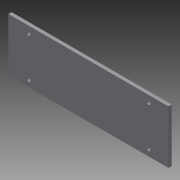
# Autodesk Inventor part: Pneumatic Piston Bracket_v1
Saved by Autodesk Inventor 2013 (Build 170138000, 138)
## iProperties
Created: 2013-01-21
Part Number: Pneumatic Piston Bracket_v1
Material: Generic
Document SubType Name: Sheet Metal
Designer: motoennies
Density: 1 g/cm^3
Sheet Metal Rule: Default
Author: motoennies
Autodesk Inventor part; units mm, degrees
ref_plane "YZ Plane" through (0, 0, 0) normal (1, 0, 0) x (0, 1, 0)
ref_plane "XZ Plane" through (0, 0, 0) normal (0, 1, 0) x (-1, 0, 0)
ref_plane "XY Plane" through (0, 0, 0) normal (0, 0, 1) x (1, 0, 0)
sketch "Sketch1" plane through (0, 0, 0) normal (0, 0, 1) x (1, 0, 0)
  line L0 (0, 50.8) -> (0, 0)
  line L1 (152.4, 0) -> (152.4, 0)
  line L2 (0, 0) -> (152.4, 0)
  line L3 (152.4, 0) -> (152.4, 50.8)
  line L4 (0, 50.8) -> (152.4, 50.8)
  dimension "d23" = 50.8
  dimension "d26" = 152.4
  measures "d23" distance of L0.start L0.end
  measures "d26" distance of L0.end L1.end
extrude "Plate2" add sketch "Sketch1" along normal blind 3.048
sketch "Sketch8" plane through (0, 0, 3.048) normal (0, 0, 1) x (1, 0, 0)
  line L0 (0, 50.8) -> (120.65, 50.8) projected
  line L1 (152.4, 0) -> (0, 0) projected
  line L2 (0, 50.8) -> (19.05, 50.8)
  line L3 (19.05, 50.8) -> (19.05, 0)
  line L4 (19.05, 25.4) -> (19.05, 44.45)
  line L5 (19.05, 25.4) -> (19.05, 6.35)
  circle A0 centre (19.05, 44.45) radius 1.9844
  circle A1 centre (19.05, 6.35) radius 1.9844
  line L6 (152.4, 50.8) -> (152.4, 0) projected
  circle A2 centre (133.35, 44.45) radius 1.9812
  circle A3 centre (133.35, 6.35) radius 1.9812
  dimension "d62" = 19.05
  dimension "d63" = 19.05
  dimension "d64" = 19.05
  dimension "d65" = 3.9688
  dimension "d66" = 3.9688
  dimension "d69" = 3.9624
  dimension "d70" = 3.9624
  dimension "d71" = 19.05
  dimension "d72" = 38.1
  dimension "d73" = 19.05
  dimension "d74" = 6.35
  constraints: 8 end point, 4 centre point, 4 point on line, 2 coincident, 1 midpoint, 1 perpendicular
  measures "d62" distance of L0.start L2.end
  measures "d63" distance of L4.start L4.end
  measures "d64" distance of L4.start L5.end
  measures "d65" diameter of A0
  measures "d66" diameter of A1
  measures "d69" diameter of A2
  measures "d70" diameter of A3
  measures "d71" distance from line of L6 A2.centre
  measures "d72" distance of A2.centre A3.centre
  measures "d73" distance from line of L6 A3.centre
  measures "d74" distance from line of L1 A3.centre
extrude "Cut5" cut sketch "Sketch8" against normal blind 3.048
equation "\"d75\" = Thickness"
equation "\"BendRadius\" = Thickness"
equation "\"BendReliefWidth\" = Thickness"
equation "\"BendReliefDepth\" = 0.5 * Thickness"
equation "\"CornerReliefSize\" = 4 * Thickness"
equation "\"MinimumRemnant\" = 2 * Thickness"
equation "\"TransitionRadius\" = BendRadius"
equation "\"JacobiRadiusSize\" = BendRadius"
equation "\"GapSize\" = Thickness"
equation "\"d10\" = BendRadius"
equation "\"d11\" = BendRadius"
equation "\"Thickness\" = 3.048"
body "Solid2"
